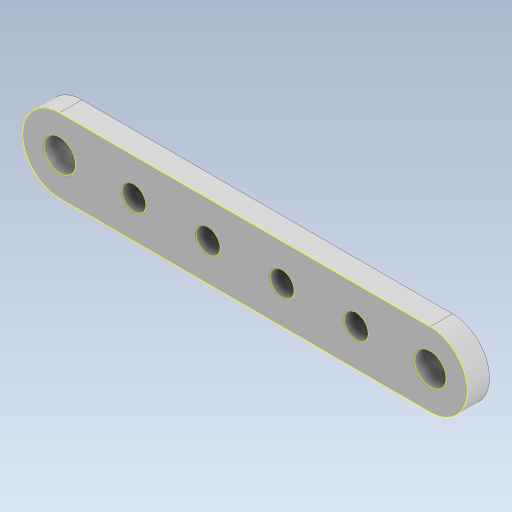
# Autodesk Inventor part: 零件12
Saved by Autodesk Inventor 2023 (Build 270158000, 158)
## iProperties
Created: 2023-04-16
Part Number: 零件12
Material: 一般
Document SubType Name: Modeling
Designer: JOU
Density: 1 g/cm^3
Appearance: 預設
Author: JOU
Autodesk Inventor part; units mm, degrees
ref_plane "YZ Plane" through (0, 0, 0) normal (1, 0, 0) x (0, 1, 0)
ref_plane "XZ Plane" through (0, 0, 0) normal (0, 1, 0) x (-1, 0, 0)
ref_plane "XY Plane" through (0, 0, 0) normal (0, 0, 1) x (1, 0, 0)
sketch "草圖1" plane through (0, 0, 0) normal (0, 0, 1) x (1, 0, 0)
  line L0 (-50, 0) -> (0, 0) construction
  line L1 (-50, -5) -> (0, -5)
  line L2 (0, 5) -> (-50, 5)
  arc A0 (-50, 5) -> (-50, -5) centre (-50, 0) ccw
  arc A1 (0, -5) -> (0, 5) centre (0, 0) ccw
  circle A2 centre (-50, 0) radius 2.1
  circle A3 centre (0, 0) radius 2.1
  circle A4 centre (-40, 0) radius 1.6
  circle A5 centre (-30, 0) radius 1.6
  circle A6 centre (-20, 0) radius 1.6
  circle A7 centre (-10, 0) radius 1.6
  point P0 (-25, 0)
  dimension "d0" = 50
  dimension "d1" = 10
  dimension "d2" = 4.2
  dimension "d3" = 4.2
  dimension "d4" = 3.2
  dimension "d11" = 3.2
  dimension "d12" = 10
  dimension "d13" = 10
  dimension "d16" = 10
  constraints: 8 centre point, 8 end point, 4 point on circle, 4 tangent, 3 coincident, 2 horizontal, 2 point on line, 1 midpoint, 1 parallel, 4 other
  measures "d0" distance of L2.start L2.end
  measures "d1" distance between parallel lines of L1 L2
  measures "d2" diameter of A2
  measures "d3" diameter of A3
  measures "d4" diameter of A4
  measures "d11" diameter of A5
  measures "d12" distance of L0.start A4.centre
  measures "d13" distance of A5.centre A4.centre
  measures "d16" distance of A5.centre A6.centre
extrude "擠出1" add sketch "草圖1" along normal blind 3
sketch "草圖3" plane through (0, 0, 3) normal (0, 0, 1) x (1, 0, 0)
  arc A0 (0, -5) -> (0, 5) centre (0, 0) ccw projected
  line L0 (0, 5) -> (-50, 5) projected
  arc A1 (-50, 5) -> (-50, -5) centre (-50, 0) ccw projected
  line L1 (-50, -5) -> (0, -5) projected
  circle A2 centre (-40, 0) radius 1.6 projected
  circle A3 centre (-30, 0) radius 1.6 projected
  circle A4 centre (-20, 0) radius 1.6 projected
  circle A5 centre (-10, 0) radius 1.6 projected
  circle A6 centre (0, 0) radius 2.1 projected
  circle A7 centre (-50, 0) radius 2.1 projected
